Stand+shape (Autodesk Fusion 360 design; units mm, degrees)
part number: 2025-10-23-21-49-31-248
Autodesk Fusion 360 part; units mm, degrees
note: some values were not read from the file. Set by a fixed rule: which face or edge a step refers to.
sketch "Sketch1" plane through (0, 0, 0) normal (0, 0, 1) x (1, 0, 0)
  line L0 (0, 101.6) -> (50.8, 101.6)
  line L1 (50.8, 101.6) -> (50.8, 0)
  line L2 (50.8, 0) -> (0, 0)
  line L3 (0, 0) -> (0, 101.6)
  line L4 (0, 622.3) -> (50.8, 622.3)
  line L5 (50.8, 622.3) -> (50.8, 723.9)
  line L6 (50.8, 723.9) -> (0, 723.9)
  line L7 (0, 723.9) -> (0, 622.3)
  line L8 (1346.2, 0) -> (1397, 0)
  line L9 (1397, 0) -> (1397, 101.6)
  line L10 (1397, 101.6) -> (1346.2, 101.6)
  line L11 (1346.2, 101.6) -> (1346.2, 0)
  line L12 (1346.2, 723.9) -> (1397, 723.9)
  line L13 (1397, 723.9) -> (1397, 622.3)
  line L14 (1397, 622.3) -> (1346.2, 622.3)
  line L15 (1346.2, 622.3) -> (1346.2, 723.9)
  constraint horizontal L0
  constraint vertical L1
  constraint horizontal L2
  constraint vertical L3
  constraint horizontal L4
  constraint vertical L5
  constraint horizontal L6
  constraint vertical L7
  constraint horizontal L8
  constraint vertical L9
  constraint horizontal L10
  constraint vertical L11
  constraint horizontal L12
  constraint vertical L13
  constraint horizontal L14
  constraint vertical L15
extrude "Extrude1" add sketch "Sketch1" along normal blind 1219.2 makes body 1 at (50.8, 67.7333, 406.4) makes body 2 at (1397, 690.0333, 406.4) makes body 3 at (0, 690.0333, 406.4) makes body 4 at (1346.2, 67.7333, 406.4)
sketch "Sketch2" plane through (0, 622.3, 0) normal (0, -1, 0) x (1, 0, 0)
  line L0 (0, 0) -> (50.8, 0)
  line L1 (50.8, 0) -> (50.8, 1219.2)
  line L2 (50.8, 1219.2) -> (0, 1219.2)
  line L3 (0, 1219.2) -> (0, 0)
  line L4 (0, 1219.2) -> (50.8, 1219.2)
  line L5 (50.8, 1219.2) -> (50.8, 1117.6)
  line L6 (50.8, 1117.6) -> (0, 1117.6)
  line L7 (0, 1117.6) -> (0, 1219.2)
  line L8 (1346.2, 1219.2) -> (1397, 1219.2)
  line L9 (1397, 1219.2) -> (1397, 1117.6)
  line L10 (1397, 1117.6) -> (1346.2, 1117.6)
  line L11 (1346.2, 1117.6) -> (1346.2, 1219.2)
  constraint horizontal L4
  constraint vertical L5
  constraint horizontal L6
  constraint vertical L7
  constraint coincident L1 L5.end
  constraint coincident L2.end L3.start
  constraint horizontal L8
  constraint vertical L9
  constraint horizontal L10
  constraint vertical L11
extrude "Extrude2" add sketch "Sketch2" along normal blind 520.7 contours L1 L2 L3 L4 L5 L6 L7 | L8 L9 L10 L11 bodies 1 2 3 4
sketch "Sketch3" plane through (1346.2, 0, 0) normal (-1, 0, 0) x (0, -1, 0)
  line L0 (-723.9, 0) -> (-622.3, 0)
  line L1 (-622.3, 0) -> (-622.3, 1117.6)
  line L2 (-622.3, 1117.6) -> (-101.6, 1117.6)
  line L3 (-101.6, 1117.6) -> (-101.6, 0)
  line L4 (-101.6, 0) -> (0, 0)
  line L5 (0, 0) -> (0, 1219.2)
  line L6 (0, 1219.2) -> (-101.6, 1219.2)
  line L7 (-101.6, 1219.2) -> (-622.3, 1219.2)
  line L8 (-622.3, 1219.2) -> (-723.9, 1219.2)
  line L9 (-723.9, 1219.2) -> (-723.9, 0)
  line L10 (-101.6, 1219.2) -> (0, 1219.2)
  line L11 (0, 1219.2) -> (0, 1168.4)
  line L12 (0, 1168.4) -> (-101.6, 1168.4)
  line L13 (-101.6, 1168.4) -> (-101.6, 1219.2)
  line L14 (-723.9, 1219.2) -> (-622.3, 1219.2)
  line L15 (-622.3, 1219.2) -> (-622.3, 1168.4)
  line L16 (-622.3, 1168.4) -> (-723.9, 1168.4)
  line L17 (-723.9, 1168.4) -> (-723.9, 1219.2)
  constraint horizontal L10
  constraint vertical L11
  constraint horizontal L12
  constraint vertical L13
  constraint coincident L5 L11.end
  constraint coincident L6.end L7.start
  constraint horizontal L14
  constraint vertical L15
  constraint horizontal L16
  constraint vertical L17
  constraint coincident L8.end L9.start
extrude "Extrude3" cut sketch "Sketch3" along normal blind 1295.4 contours L8 L9 L14 L15 L16 L17 | L5 L6 L10 L11 L12 L13 bodies 1
sketch "Sketch4" plane through (50.8, 0, 0) normal (1, 0, 0) x (0, 1, 0)
  line L0 (0, 0) -> (101.6, 0)
  line L1 (101.6, 0) -> (101.6, 1117.6)
  line L2 (101.6, 1117.6) -> (622.3, 1117.6)
  line L3 (622.3, 1117.6) -> (622.3, 0)
  line L4 (622.3, 0) -> (723.9, 0)
  line L5 (723.9, 0) -> (723.9, 1219.2)
  line L6 (723.9, 1219.2) -> (101.6, 1219.2)
  line L7 (101.6, 1219.2) -> (0, 1219.2)
  line L8 (0, 1219.2) -> (0, 0)
  line L9 (0, 1219.2) -> (50.8, 1219.2)
  line L10 (50.8, 1219.2) -> (50.8, 1117.6)
  line L11 (50.8, 1117.6) -> (0, 1117.6)
  line L12 (0, 1117.6) -> (0, 1219.2)
  line L13 (723.9, 1219.2) -> (673.1, 1219.2)
  line L14 (673.1, 1219.2) -> (673.1, 1117.6)
  line L15 (673.1, 1117.6) -> (723.9, 1117.6)
  line L16 (723.9, 1117.6) -> (723.9, 1219.2)
  constraint horizontal L9
  constraint vertical L10
  constraint horizontal L11
  constraint vertical L12
  constraint coincident L7.end L8.start
  constraint horizontal L13
  constraint vertical L14
  constraint horizontal L15
  constraint vertical L16
  constraint coincident L5.end L6.start
extrude "Extrude4" add sketch "Sketch4" along normal blind 1295.4 contours L7 L8 L9 L10 L11 L12 | L5 L6 L13 L14 L15 L16 bodies 1 2
sketch "Sketch5" plane through (0, 0, 1219.2) normal (0, 0, 1) x (-1, 0, 0)
  line L0 (-1346.2, 0) -> (-1397, 0)
  line L1 (-1397, 0) -> (-1397, -101.6)
  line L2 (-1397, -101.6) -> (-1397, -622.3)
  line L3 (-1397, -622.3) -> (-1397, -723.9)
  line L4 (-1397, -723.9) -> (-1346.2, -723.9)
  line L5 (-1346.2, -723.9) -> (0, -723.9)
  line L6 (0, -723.9) -> (0, -101.6)
  line L7 (0, -101.6) -> (0, 0)
  line L8 (0, 0) -> (-1346.2, 0)
  line L9 (-1346.2, -50.8) -> (-50.8, -50.8)
  line L10 (-50.8, -50.8) -> (-50.8, -101.6)
  line L11 (-50.8, -101.6) -> (-50.8, -673.1)
  line L12 (-50.8, -673.1) -> (-1346.2, -673.1)
  line L13 (-1346.2, -673.1) -> (-1346.2, -622.3)
  line L14 (-1346.2, -622.3) -> (-1346.2, -101.6)
  line L15 (-1346.2, -101.6) -> (-1346.2, -50.8)
  line L16 (-736.6, 0) -> (-660.4, 0)
  line L17 (-660.4, 0) -> (-660.4, -723.9)
  line L18 (-660.4, -723.9) -> (-736.6, -723.9)
  line L19 (-736.6, -723.9) -> (-736.6, 0)
  dimension "d9" = 76.2
  constraint horizontal L16
  constraint vertical L17
  constraint horizontal L18
  constraint vertical L19
  constraint coincident L8 L16.start
  measures "d9" distance of L16.start L16.end
extrude "Extrude5" add sketch "Sketch5" along normal blind 6.35 separate body contours L8 L9 L16 L17 L19 | L9 L12 L17 L19 | L5 L12 L17 L18 L19 makes body 5
sketch "Sketch6" plane through (0, 0, 1225.55) normal (0, 0, 1) x (-1, 0, 0)
  line L0 (-736.6, -723.9) -> (-660.4, -723.9)
  line L1 (-660.4, -723.9) -> (-660.4, 0)
  line L2 (-660.4, 0) -> (-736.6, 0)
  line L3 (-736.6, 0) -> (-736.6, -723.9)
  line L4 (-685.8, -330.2) -> (-711.2, -330.2)
  line L5 (-711.2, -330.2) -> (-711.2, -355.6)
  line L6 (-711.2, -355.6) -> (-685.8, -355.6)
  line L7 (-685.8, -355.6) -> (-685.8, -330.2)
  line L8 (-685.7427, -361.95) -> (-711.2, -361.95)
  line L9 (-711.2, -361.95) -> (-711.2, -336.55)
  line L10 (-711.2, -336.55) -> (-685.7427, -336.55)
  line L11 (-685.7427, -336.55) -> (-685.7427, -361.95)
  dimension "d12" = 25.4
  constraint horizontal L4
  constraint vertical L5
  constraint horizontal L6
  constraint vertical L7
  constraint horizontal L8
  constraint vertical L9
  constraint horizontal L10
  constraint vertical L11
  measures "d12" distance of L8.start L10.end
sketch "Sketch7" plane through (0, 0, 1225.55) normal (0, 0, 1) x (-1, 0, 0)
  line L0 (-685.8, -374.65) -> (-711.2, -374.65)
  line L1 (-711.2, -374.65) -> (-711.2, -349.25)
  line L2 (-711.2, -349.25) -> (-685.8, -349.25)
  line L3 (-685.8, -349.25) -> (-685.8, -374.65)
  constraint horizontal L0
  constraint vertical L1
  constraint horizontal L2
  constraint vertical L3
extrude "Extrude6" cut sketch "Sketch7" against normal blind 6.35 bodies 5
sketch "Sketch8" plane through (0, 0, 1225.55) normal (0, 0, 1) x (-1, 0, 0)
  line L0 (-679.45, -381) -> (-717.55, -381)
  line L1 (-717.55, -381) -> (-717.55, -374.65)
  line L2 (-717.55, -374.65) -> (-679.45, -374.65)
  line L3 (-679.45, -374.65) -> (-679.45, -381)
  line L4 (-679.45, -374.65) -> (-685.8, -374.65)
  line L5 (-685.8, -374.65) -> (-685.8, -342.9)
  line L6 (-685.8, -342.9) -> (-679.45, -342.9)
  line L7 (-679.45, -342.9) -> (-679.45, -374.65)
  line L8 (-685.8, -342.9) -> (-717.55, -342.9)
  line L9 (-717.55, -342.9) -> (-717.55, -349.25)
  line L10 (-717.55, -349.25) -> (-685.8, -349.25)
  line L11 (-685.8, -349.25) -> (-685.8, -342.9)
  line L12 (-717.55, -349.25) -> (-711.2, -349.25)
  line L13 (-711.2, -349.25) -> (-711.2, -374.65)
  line L14 (-711.2, -374.65) -> (-717.55, -374.65)
  line L15 (-717.55, -374.65) -> (-717.55, -349.25)
  constraint horizontal L0
  constraint vertical L1
  constraint horizontal L2
  constraint vertical L3
  constraint horizontal L4
  constraint vertical L5
  constraint horizontal L6
  constraint vertical L7
  constraint horizontal L8
  constraint vertical L9
  constraint horizontal L10
  constraint vertical L11
  constraint horizontal L12
  constraint vertical L13
  constraint horizontal L14
  constraint vertical L15
  constraint coincident L2 L13.end
extrude "Extrude7" cut sketch "Sketch8" against normal blind 6.35 contours L0 L1 L2 L3 L4 L14 | L2 L4 L5 L6 L7 L11 | L2 L10 L12 L13 L14 L15 | L5 L8 L9 L10 L11 L12 bodies 5
sketch "Sketch9" plane through (1397, 0, 0) normal (1, 0, 0) x (0, 1, 0)
  line L0 (622.3, 0) -> (723.9, 0)
  line L1 (723.9, 0) -> (723.9, 1219.2)
  line L2 (723.9, 1219.2) -> (622.3, 1219.2)
  line L3 (622.3, 1219.2) -> (101.6, 1219.2)
  line L4 (101.6, 1219.2) -> (0, 1219.2)
  line L5 (0, 1219.2) -> (0, 0)
  line L6 (0, 0) -> (101.6, 0)
  line L7 (101.6, 0) -> (101.6, 1117.6)
  line L8 (101.6, 1117.6) -> (622.3, 1117.6)
  line L9 (622.3, 1117.6) -> (622.3, 0)
  line L10 (50.8, 1168.4) -> (673.1, 1168.4)
  line L11 (673.1, 1168.4) -> (673.1, 0)
  line L12 (673.1, 0) -> (50.8, 0)
  line L13 (50.8, 0) -> (50.8, 1168.4)
  constraint horizontal L10
  constraint vertical L11
  constraint horizontal L12
  constraint vertical L13
  constraint midpoint L0 L11.end
extrude "Extrude8" cut sketch "Sketch9" against normal blind 50.8 contours L0 L6 L7 L8 L9 L10 L11 L12 L13 bodies 1
sketch "Sketch10" plane through (0, 723.9, 0) normal (0, 1, 0) x (-1, 0, 0)
  line L0 (-50.8, 0) -> (0, 0)
  line L1 (0, 0) -> (0, 1219.2)
  line L2 (0, 1219.2) -> (-1346.2, 1219.2)
  line L3 (-1346.2, 1219.2) -> (-1397, 1219.2)
  line L4 (-1397, 1219.2) -> (-1397, 0)
  line L5 (-1397, 0) -> (-1346.2, 0)
  line L6 (-1346.2, 0) -> (-1346.2, 1117.6)
  line L7 (-1346.2, 1117.6) -> (-50.8, 1117.6)
  line L8 (-50.8, 1117.6) -> (-50.8, 0)
  line L9 (-1346.2, 1168.4) -> (-50.8, 1168.4)
  line L10 (-50.8, 1168.4) -> (-50.8, 1117.6)
  line L11 (-50.8, 1117.6) -> (-1346.2, 1117.6)
  line L12 (-1346.2, 1117.6) -> (-1346.2, 1168.4)
  constraint horizontal L9
  constraint vertical L10
  constraint horizontal L11
  constraint vertical L12
  constraint coincident L7.end L8.start
extrude "Extrude9" cut sketch "Sketch10" against normal blind 50.8 contours L7 L9 L10 L11 L12 bodies 1
sketch "Sketch11" plane through (0, 0, 0) normal (-1, 0, 0) x (0, -1, 0)
  line L0 (-101.6, 0) -> (0, 0)
  line L1 (0, 0) -> (0, 1219.2)
  line L2 (0, 1219.2) -> (-101.6, 1219.2)
  line L3 (-101.6, 1219.2) -> (-723.9, 1219.2)
  line L4 (-723.9, 1219.2) -> (-723.9, 0)
  line L5 (-723.9, 0) -> (-622.3, 0)
  line L6 (-622.3, 0) -> (-622.3, 1117.6)
  line L7 (-622.3, 1117.6) -> (-101.6, 1117.6)
  line L8 (-101.6, 1117.6) -> (-101.6, 0)
  line L9 (-50.8, 1168.4) -> (-673.1, 1168.4)
  line L10 (-673.1, 1168.4) -> (-673.1, 0)
  line L11 (-673.1, 0) -> (-50.8, 0)
  line L12 (-50.8, 0) -> (-50.8, 1168.4)
  constraint horizontal L9
  constraint vertical L10
  constraint horizontal L11
  constraint vertical L12
  constraint midpoint L5 L10.end
extrude "Extrude10" cut sketch "Sketch11" against normal blind 50.8 contours L0 L5 L6 L7 L8 L9 L10 L11 L12 bodies 1
sketch "Sketch12" plane through (0, 0, 0) normal (0, -1, 0) x (1, 0, 0)
  line L0 (1346.2, 0) -> (1397, 0)
  line L1 (1397, 0) -> (1397, 1219.2)
  line L2 (1397, 1219.2) -> (1346.2, 1219.2)
  line L3 (1346.2, 1219.2) -> (0, 1219.2)
  line L4 (0, 1219.2) -> (0, 0)
  line L5 (0, 0) -> (50.8, 0)
  line L6 (50.8, 0) -> (50.8, 1117.6)
  line L7 (50.8, 1117.6) -> (1346.2, 1117.6)
  line L8 (1346.2, 1117.6) -> (1346.2, 0)
  line L9 (50.8, 1168.4) -> (1346.2, 1168.4)
  line L10 (1346.2, 1168.4) -> (1346.2, 1117.6)
  line L11 (1346.2, 1117.6) -> (50.8, 1117.6)
  line L12 (50.8, 1117.6) -> (50.8, 1168.4)
  constraint horizontal L9
  constraint vertical L10
  constraint horizontal L11
  constraint vertical L12
  constraint coincident L7.end L8.start
extrude "Extrude11" cut sketch "Sketch12" against normal blind 50.8 contours L7 L9 L10 L11 L12 bodies 1
move_face "MoveFace1" by (0, 0, -12.7) 4 faces at (914.4, 16.9333, 1219.2) (1380.0666, 622.3, 1219.2) (1363.1333, 101.6, 1219.2) (1363.1333, 275.1667, 1219.2) on bodies 1
move_face "MoveFace2" by (-12.7, 0, 0) 1 faces at (1397, 706.9667, 791.6333) on bodies 1
move_face "MoveFace3" by (12.7, 0, 0) 1 faces at (0, 16.9333, 791.6333) on bodies 1
move_face "MoveFace4" by (0, 12.7, 0) 1 faces at (1371.6, 0, 774.7) on bodies 1
move_face "MoveFace5" by (0, -12.7, 0) 1 faces at (482.6, 723.9, 1193.8) on bodies 1
